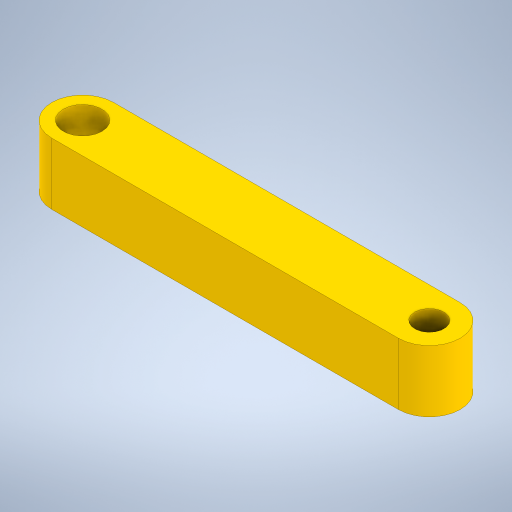
# Autodesk Inventor part: Motor to Shaft Connection for Side to Side motion
Saved by Autodesk Inventor 2023.1 (Build 271208000, 208)
## iProperties
Created: 2022-12-21
Part Number: Motor to Shaft Connection for Side to Side motion
Material: Generic
Document SubType Name: Modeling
Designer: shubh
Density: 1 g/cm^3
Appearance: Default(1)
Author: shubh
Autodesk Inventor part; units mm, degrees
ref_plane "YZ Plane" through (0, 0, 0) normal (1, 0, 0) x (0, 1, 0)
ref_plane "XZ Plane" through (0, 0, 0) normal (0, 1, 0) x (-1, 0, 0)
ref_plane "XY Plane" through (0, 0, 0) normal (0, 0, 1) x (1, 0, 0)
sketch "Sketch1" plane through (0, 0, 0) normal (0, 1, 0) x (-1, 0, 0)
  circle A0 centre (63.3603, 0) radius 3.9751
  circle A1 centre (-7.9375, 0) radius 3
  line L0 (63.3603, 6.35) -> (-7.9375, 6.35)
  line L1 (-7.9375, -6.35) -> (63.3603, -6.35)
  arc A2 (63.3603, -6.35) -> (63.3603, 6.35) centre (63.3603, 0) ccw
  arc A3 (-7.9375, 6.35) -> (-7.9375, -6.35) centre (-7.9375, 0) ccw
  point P0 (0, 0)
  dimension "d0" = 7.9502
  dimension "d1" = 6
  dimension "d3" = 12.7
  dimension "d4" = 12.7
  dimension "d7" = 71.2978
  constraints: 4 centre point, 4 end point, 4 point on circle, 2 coincident, 1 horizontal, 1 parallel
  measures "d0" diameter of A0
  measures "d1" diameter of A1
  measures "d3" diameter of A2
  measures "d4" diameter of A3
  measures "d7" distance of L1.start L1.end
extrude "Extrusion1" add sketch "Sketch1" along normal blind 12.7
body "Solid1"
